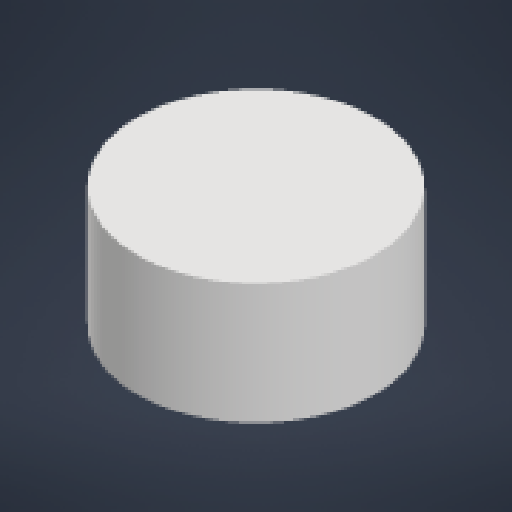
# Autodesk Inventor part: MiddleJointCylinder
Saved by Autodesk Inventor 2026.2 (Build 302298010, 298A)
## iProperties
Created: 2026-06-25
Part Number: MiddleJointCylinder
Material: Generic
Document SubType Name: Modeling
Designer: frede
Density: 1 g/cm^3
Appearance: Default
Author: frede
Autodesk Inventor part; units mm, degrees
ref_plane "YZ Plane" through (0, 0, 0) normal (1, 0, 0) x (0, 1, 0)
ref_plane "XZ Plane" through (0, 0, 0) normal (0, 1, 0) x (-1, 0, 0)
ref_plane "XY Plane" through (0, 0, 0) normal (0, 0, 1) x (1, 0, 0)
sketch "Sketch1" plane through (0, 0, 0) normal (0, 1, 0) x (-1, 0, 0)
  circle A0 centre (0, 0) radius 4.925
  dimension "d0" = 9.85
  constraints: 1 centre point, 1 coincident
  measures "d0" diameter of A0
extrude "Extrusion1" add sketch "Sketch1" along normal blind 5
sketch "Sketch2" plane through (0, 0, 0) normal (1, 0, 0) x (0, 1, 0)
  line L0 (5, -4.925) -> (5, 4.925) projected
  line L1 (0, -4.925) -> (0, 4.925) projected
  line L2 (5, 0) -> (0, 0)
  circle A0 centre (2.5, 0) radius 1.5
  dimension "d3" = 3
  constraints: 2 end point, 2 midpoint, 1 centre point, 1 horizontal
  measures "d3" diameter of A0
extrude "Extrusion2" cut sketch "Sketch2" along normal mid plane 20
fillet "Fillet1" radius 2 2 edges at (4.925, 5, 0) (4.925, 0, 0)
sketch "Sketch3" plane through (0, 0, 0) normal (0, 0, 1) x (1, 0, 0)
  line L0 (4.7176, 2) -> (-4.7176, 2) projected
  line L1 (-4.7176, 3) -> (4.7176, 3) projected
  line L2 (0, 3) -> (0, 2)
  circle A0 centre (0, 2.5) radius 1.5
  point P0 (0, 0)
  dimension "d7" = 3
  constraints: 3 midpoint, 2 end point, 2 vertical alignment, 1 centre point
  measures "d7" diameter of A0
extrude "Extrusion3" cut sketch "Sketch3" along normal mid plane 20
sketch "Sketch4" plane through (0, 5, 0) normal (0, 1, 0) x (1, 0, 0)
  line L0 (0, 0) -> (1.5, -1.5) projected
  line L1 (-1.5, 1.5) -> (1.5, 1.5)
  line L2 (1.5, 1.5) -> (1.5, -1.5)
  line L3 (1.5, -1.5) -> (-1.5, -1.5)
  line L4 (-1.5, -1.5) -> (-1.5, 1.5)
  line L5 (-1.5, 1.5) -> (1.5, -1.5) construction
  line L6 (1.5, 1.5) -> (-1.5, -1.5) construction
  constraints: 12 end point, 2 midpoint, 2 parallel, 1 horizontal, 1 perpendicular
extrude "Extrusion4" add sketch "Sketch4" against normal up to surface (5 mm away)
body "Solid1"
